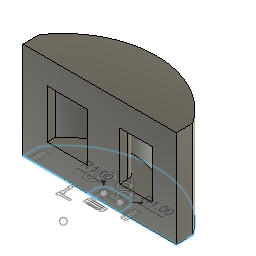
filler (Autodesk Fusion 360 design; units mm, degrees)
Autodesk Fusion 360 part; units mm, degrees
note: some values were not read from the file. Set by a fixed rule: which face or edge a step refers to.
sketch "Sketch1" plane through (0, 0, 0) normal (0, 0, 1) x (1, 0, 0) in component "Component"
  arc A0 (19, 12) -> (0, 12) centre (9.5, 5.5) ccw
  line L0 (19, 10) -> (19, 12)
  line L1 (0, 10) -> (0, 12)
  line L2 (0, 10) -> (19, 10)
  line L3 (8, 10) -> (12, 10)
  line L4 (12, 10) -> (12, 11)
  line L5 (11, 12) -> (9, 12)
  line L6 (8, 11) -> (8, 10)
  arc A1 (9, 12) -> (8, 11) centre (9, 11) ccw
  arc A2 (12, 11) -> (11, 12) centre (11, 11) ccw
  dimension "d27" = 1
  dimension "d28" = 1
  constraint vertical L1
  constraint horizontal L2
  constraint horizontal L3
  constraint vertical L4
  constraint horizontal L5
  constraint vertical L6
  constraint coincident L2 L3.start
  constraint tangent L5 A1
  constraint tangent L6 A1
  constraint tangent L4 A2
  constraint tangent L5 A2
  measures "d27" radius of A1
  measures "d28" radius of A2
extrude "Extrude4" add sketch "Sketch1" along normal blind 12 makes body 1 in component "Component"
extrude "Extrude4'" add sketch "Sketch1" along normal blind 12 separate body makes body 2
shell "Shell1" thickness 3 removed faces 3 at (2.6667, 10, 4) at (9.3333, 10, 4) at (14.3333, 10, 4) on bodies 2
shell "Shell1'" thickness 3 removed faces 3 at (2.6667, 10, 4) at (9.3333, 10, 4) at (14.3333, 10, 4) on bodies 1 in component "Component"
extrude "Extrude5" add sketch "Sketch1" along normal blind 12 separate body contours L2 L3 L4 L5 L6 A1 A2 makes body 3 in component "Component"
extrude "Extrude6" add sketch "Sketch1" along normal blind 12 contours L2 L3 L4 L5 L6 A1 A2 bodies 1 3 in component "Component"
extrude "Extrude3" [suppressed] in component "Component"
component "Component" placed x (1, 0, 0) y (0, 1, 0) z (0, 0, 1) at (0, 0, 0)
